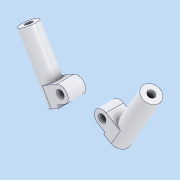
# Autodesk Inventor part: GripperCompensatorLeft
Saved by Autodesk Inventor 2020.2 (Build 242310000, 310)
## iProperties
Created: 2020-03-14
Part Number: GripperCompensatorLeft
Material: Generisch
Document SubType Name: Modeling
Designer: JochenAlt
Density: 1 g/cm^3
Appearance: Vorgabe
Author: JochenAlt
Autodesk Inventor part; units mm, degrees
ref_plane "YZ Plane" through (0, 0, 0) normal (1, 0, 0) x (0, 1, 0)
ref_plane "XZ Plane" through (0, 0, 0) normal (0, 1, 0) x (-1, 0, 0)
ref_plane "XY Plane" through (0, 0, 0) normal (0, 0, 1) x (1, 0, 0)
derived "Centre.ipt"
sketch "MainConstruction" plane through (0, 0, 0) normal (0, 0, 1) x (1, 0, 0)
  line L0 (-44.4573, 0) -> (45.9096, 0) construction
  line L1 (0, -41.3) -> (0, 41.3) construction
  line L2 (-12, 16.3923) -> (12, 16.3923) construction
  line L3 (20.547, 2.8038) -> (8.1962, -18.5885) construction
  line L4 (-8.1962, -18.5885) -> (-11.1962, -13.3923) construction
  line L5 (0, -16.3923) -> (24, -16.3923) construction
  line L6 (0, -16.3923) -> (-24, -16.3923) construction
  line L7 (6, -16.3923) -> (6, -10.3923) construction
  line L8 (6, -10.3923) -> (11.1962, -13.3923) construction
  line L9 (8.1962, -18.5885) -> (11.1962, -13.3923) construction
  line L10 (0, -16.3923) -> (6, -16.3923) construction
  line L11 (-6, -10.3923) -> (-6, -16.3923) construction
  line L12 (-6, -10.3923) -> (-11.1962, -13.3923) construction
  line L13 (0, 16.3923) -> (0, 0) construction
  line L14 (0, 0) -> (0, -16.3923) construction
  line L15 (-12, 14.3923) -> (12, 14.3923) construction
  line L16 (-12, 16.3923) -> (-12, 14.3923) construction
  line L17 (-12, 27) -> (12, 27) construction
  line L18 (-29.3827, -3.1077) -> (-17.3827, -23.8923) construction
  line L19 (0, 16.3923) -> (0, 27) construction
  line L20 (-23.3827, -13.5) -> (-14.1962, -8.1962) construction
  arc A0 (-2.6277, -14.0839) -> (-3.3698, -6.14) centre (-6, -10.3923) ccw construction
  arc A1 (3.3698, -6.14) -> (2.6277, -14.0839) centre (6, -10.3923) ccw construction
  line L21 (-27.2176, -1.8577) -> (-31.5477, -4.3577) construction
  line L22 (-15.2176, -22.6423) -> (-19.5477, -25.1423) construction
  line L23 (19.5477, -25.1423) -> (15.2176, -22.6423) construction
  circle A2 centre (0, 0) radius 22 construction
  line L24 (12, 14.3923) -> (12, 16.3923) construction
  line L25 (23.3827, -13.5) -> (14.1962, -8.1962) construction
  line L26 (20.1962, 2.1962) -> (14.1962, -8.1962) construction
  line L27 (11.1962, -13.3923) -> (14.1962, -8.1962) construction
  line L28 (-6, -16.3923) -> (0, -16.3923) construction
  line L29 (8.1962, -18.5885) -> (15.2176, -22.6423) construction
  line L30 (-15.2176, -22.6423) -> (-8.1962, -18.5885) construction
  line L31 (-12, 29.5) -> (-12, 24.5) construction
  line L32 (12, 29.5) -> (12, 24.5) construction
  line L33 (12, 24.5) -> (12, 16.3923) construction
  line L34 (-12, 24.5) -> (-12, 16.3923) construction
  line L35 (-11.1962, -13.3923) -> (-8.1962, -18.5885) construction
  line L36 (-11.1962, -13.3923) -> (-20.1962, 2.1962) construction
  line L37 (27.2176, -1.8577) -> (31.5477, -4.3577) construction
  line L38 (17.3827, -23.8923) -> (29.3827, -3.1077) construction
  line L39 (27.2176, -1.8577) -> (21.9687, 1.1728) construction
  line L40 (-27.2176, -1.8577) -> (-21.9687, 1.1728) construction
  line L41 (20.1962, 2.1962) -> (21.9687, 1.1728) construction
  line L42 (-21.9687, 1.1728) -> (-20.1962, 2.1962) construction
  line L43 (0, -16.3923) -> (0, -24.5) construction
  line L44 (0, -24.5) -> (0, -29.5) construction
  line L45 (0, -27) -> (24, -27) construction
  line L46 (18.4641, 3.1962) -> (6.4641, -17.5885) construction
  line L47 (-18.4641, 3.1962) -> (-6.4641, -17.5885) construction
  line L48 (-20.1962, 2.1962) -> (-18.4641, 3.1962) construction
  line L49 (20.1962, 2.1962) -> (18.4641, 3.1962) construction
  line L50 (3.3698, -6.14) -> (18.4641, 3.1962) construction
  line L51 (-18.4641, 3.1962) -> (-3.3698, -6.14) construction
  circle A3 centre (30.5, 27) radius 2.5 construction
  line L52 (12, 14.3923) -> (16.25, 14.3923) construction
  line L53 (16.25, 14.3923) -> (31.8962, 24.9262) construction
  line L54 (29.1038, 29.0738) -> (10.2677, 16.3923) construction
  line L55 (12, 16.3923) -> (10.2677, 16.3923) construction
  line L56 (8.1962, -18.5885) -> (6.4641, -17.5885) construction
  line L57 (6.4641, -17.5885) -> (2.6277, -14.0839) construction
  line L58 (-8.1962, -18.5885) -> (-6.4641, -17.5885) construction
  line L59 (-6.4641, -17.5885) -> (-2.6277, -14.0839) construction
  line L60 (4.7294, -16.5869) -> (6.4641, -17.5885) construction
sketch "Skizze2" plane through (0, 0, 0) normal (0, 0, 1) x (1, 0, 0)
  line L0 (-44.4573, 0) -> (45.9096, 0) construction
  line L1 (0, -41.3) -> (0, 41.3) construction
  line L2 (20.547, 2.8038) -> (8.1962, -18.5885) construction
  line L3 (-12, 16.3923) -> (12, 16.3923) construction
  line L4 (0, -16.3923) -> (24, -16.3923) construction
  line L5 (0, -16.3923) -> (-24, -16.3923) construction
  circle A0 centre (-6, -10.3923) radius 1.1
  arc A1 (-4.875, -12.3409) -> (-7.125, -8.4437) centre (-6, -10.3923) ccw
  line L6 (-15.4486, 1.4731) -> (-19.7787, -1.0269)
  line L7 (-15.4486, 1.4731) -> (-6.8236, -13.4659)
  line L8 (-19.7787, -1.0269) -> (-13.4037, -12.0687)
  line L9 (-7.125, -8.4437) -> (-13.4037, -12.0687)
  arc A2 (-7.9486, -11.5173) -> (-4.875, -12.3409) centre (-6, -10.3923) ccw
  line L10 (-13.4037, -12.0687) -> (-11.3613, -15.6062)
  line L11 (-23.3827, -13.5) -> (-14.1962, -8.1962) construction
  line L12 (-11.3613, -15.6062) -> (-10.7787, -16.6154)
  line L13 (-6.8236, -13.4659) -> (-6.4486, -14.1154)
  line L14 (-6.4486, -14.1154) -> (-10.7787, -16.6154)
  line L15 (-6.8236, -13.4659) -> (-4.875, -12.3409)
  line L16 (-6.8236, -13.4659) -> (-11.1537, -15.9659)
  arc A3 (-7.125, -8.4437) -> (-7.9486, -11.5173) centre (-6, -10.3923) ccw
  line L17 (-29.3827, -3.1077) -> (-17.3827, -23.8923) construction
  point P0 (0, 0)
  point P1 (6, -10.3923)
  point P2 (-9.6962, -15.9904)
  point P3 (-9.2274, -9.6576)
  point P4 (-9.0736, -9.5687)
  point P5 (-6.9774, -13.5547)
  point P6 (-20.1962, 2.1962)
  dimension "d1" = 2.2
  dimension "d2" = 4.5
  dimension "d31" = 5
  dimension "d41" = 3
  constraints: 21 end point, 7 point on circle, 6 perpendicular, 5 point on line, 4 centre point, 3 coincident, 3 tangent, 2 collinear, 2 parallel, 1 concentric, 1 other
  measures "d1" diameter of A0
  measures "d2" diameter of A1
  measures "d31" distance of L6.start L6.end
  measures "d41" distance from line of L6 point (-20.196, 2.196)
extrude "Extrusion6" add sketch "Skizze2" along normal blind 5
sketch "Profile" plane through (-18.2787, -0.1609, 0.25) normal (-0.5, 0.8660254, 0) x (0.8660254, 0.5, 0)
  circle A0 centre (0.7679, -2.25) radius 2.5
  circle A1 centre (0.7679, -2.25) radius 1
  line L0 (0.7679, 0.25) -> (0, 0.25)
  line L1 (3.2679, 0.25) -> (3.2679, -4.75) projected
  line L2 (-1.7321, 0.25) -> (-1.7321, -4.75) projected
  line L3 (3.2679, -4.75) -> (-1.7321, -4.75) projected
  line L4 (3.2679, 0.25) -> (-1.7321, 0.25) projected
  line L5 (-1.7321, 0.25) -> (-1.7321, -4.75) projected
  line L6 (-1.7321, -4.75) -> (3.2679, -4.75)
  point P0 (15.9103, 0.25)
  point P1 (-1.7321, -4.75)
  dimension "d12" = 2
  constraints: 4 end point, 4 horizontal, 2 point on line, 2 vertical, 1 centre point, 1 coincident, 1 vertical alignment, 2 other
  measures "d12" diameter of A1
extrude "Extrusion3" cut sketch "Profile" against normal through all contours A1
fillet "Rundung1" radius 2.5 5 edges at (-12.2611, -4.0478, 0) (-6.6361, -13.7906, 0) (-15.2787, -8.8212, 5) (-15.2787, -8.8212, 0) (-12.2611, -4.0478, 5)
mirror "Spiegeln1" about plane through (0, 0, 0) normal (1, 0, 0) bodies 1 separate body
